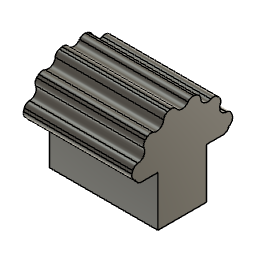
SMD-counter (Autodesk Fusion 360 archive; units mm, degrees)
design "roller"
Autodesk Fusion 360 part; units mm, degrees
note: some values were not read from the file. Set by a fixed rule: which face or edge a step refers to.
sketch "Sketch1" plane through (0, 0, 0) normal (0, 0, 1) x (1, 0, 0)
  line L0 (0, 0) -> (7.8, 0)
  line L1 (7.8, 0) -> (7.8, 3.5)
  line L2 (7.8, 3.5) -> (0, 3.5)
  line L3 (0, 3.5) -> (0, 0)
  dimension "d1" = 7.8
  dimension "d2" = 3.5
  constraint horizontal L0
  constraint vertical L1
  constraint horizontal L2
  constraint vertical L3
  constraint coincident L0.start L3.end
  measures "d1" distance of L0.start L0.end
  measures "d2" distance of L0.start L2.end
extrude "Extrude1" add sketch "Sketch1" along normal blind 3.6
sketch "Sketch2" plane through (7.8, 0, 0) normal (1, 0, 0) x (0, 1, 0)
  line L0 (0, 0) -> (3.5, 0)
  line L1 (3.5, 0) -> (3.5, 3.6)
  line L2 (3.5, 3.6) -> (0, 3.6)
  line L3 (0, 3.6) -> (0, 0)
  line L4 (-2, 3.6) -> (5.5, 3.6)
  arc A0 (5.5, 3.6) -> (-2, 3.6) centre (1.75, 3.4306) ccw
  dimension "d5" = 2
  dimension "d7" = 2
  constraint perpendicular L1 L4
  constraint collinear L2 L4
  measures "d5" distance of L3 L4.start
  measures "d7" distance of L1 L4.end
extrude "Extrude2" add sketch "Sketch2" against normal up to surface (7.8 mm away) contours L2 L4 A0
sketch "Sketch3" plane through (7.8, 0, 0) normal (1, 0, 0) x (0, 1, 0)
  line L0 (0, 0) -> (3.5, 0)
  line L1 (3.5, 0) -> (3.5, 3.6)
  line L2 (3.5, 3.6) -> (5.5, 3.6)
  arc A0 (5.5, 3.6) -> (-2, 3.6) centre (1.75, 3.4306) ccw
  line L3 (-2, 3.6) -> (0, 3.6)
  line L4 (0, 3.6) -> (0, 0)
  circle A1 centre (5.5, 3.6) radius 0.5
  circle A2 centre (4.9419, 5.4061) radius 0.5
  circle A3 centre (3.5744, 6.7112) radius 0.5
  circle A4 centre (1.7443, 7.1844) radius 0.5
  circle A5 centre (-0.0844, 6.7056) radius 0.5
  circle A6 centre (-1.4479, 5.3964) radius 0.5
  circle A7 centre (-2.0005, 3.5886) radius 0.5
  dimension "d11" = 1
  dimension "d13" = 175
  constraint coincident L2.end A0.start
  measures "d11" diameter of A1
extrude "Extrude3" cut sketch "Sketch3" against normal up to surface (7.8 mm away) contours A0 L3 A7 | L2 A0 A1 | A0 A6 | A0 A2 | A0 A5 | A0 A3 | A0 A4 picked at (-1.8378, 3.7013) picked at (5.3366, 3.7034) picked at (-1.3071, 5.3027) picked at (4.7922, 5.3274) picked at (0.0072, 6.5635) picked at (3.5029, 6.558) picked at (1.7326, 7.0157)
fillet "Fillet1" radius 0.4 14 edges at (3.9, -1.9462, 4.0856) (3.9, -1.6808, 4.9539) (3.9, -1.1583, 5.8039) (3.9, -0.5034, 6.4328) (3.9, 0.3671, 6.9204) (3.9, 1.2455, 7.1503) (3.9, 2.2432, 7.1518) (3.9, 3.1223, 6.9246) (3.9, 3.9943, 6.4396) (3.9, 4.6511, 5.8128) (3.9, 5.1762, 4.9643) (3.9, 5.4442, 4.0969) (3.9, 5, 3.6) (3.9, -1.5006, 3.6)
equation "d3 = ( 0.4 * 6 ) * 1 mm + 1.2 mm"

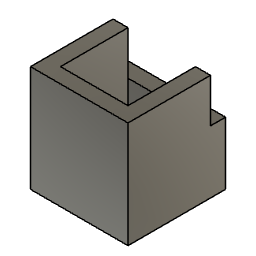
design "stopper"
Autodesk Fusion 360 part; units mm, degrees
sketch "Sketch1" plane through (0, 0, 0) normal (0, 0, 1) x (1, 0, 0)
  line L0 (0, 0) -> (7.8, 0)
  line L1 (7.8, 0) -> (7.8, 7.8)
  line L2 (7.8, 7.8) -> (0, 7.8)
  line L3 (0, 7.8) -> (0, 0)
  dimension "d1" = 7.8
  dimension "d2" = 7.8
  constraint horizontal L0
  constraint vertical L1
  constraint horizontal L2
  constraint vertical L3
  constraint coincident L0.start L3.end
  measures "d1" distance of L0.start L2.end
  measures "d2" distance of L1.end L2.end
extrude "Extrude1" add sketch "Sketch1" along normal blind 8.5
shell "Shell1" thickness 1.2 removed faces 1 at (2.6, 5.2, 8.5)
sketch "Sketch2" plane through (0, 7.8, 0) normal (0, 1, 0) x (-1, 0, 0)
  line L0 (-7.8, 0) -> (0, 0)
  line L1 (0, 0) -> (0, 8.5)
  line L2 (0, 8.5) -> (-7.8, 8.5)
  line L3 (-7.8, 8.5) -> (-7.8, 0)
  line L4 (-7.8, 8.5) -> (0, 8.5)
  line L5 (0, 8.5) -> (0, 5)
  line L6 (0, 5) -> (-7.8, 5)
  line L7 (-7.8, 5) -> (-7.8, 8.5)
  dimension "d6" = 3.5
  constraint horizontal L4
  constraint vertical L5
  constraint horizontal L6
  constraint vertical L7
  constraint coincident L1 L5.end
  constraint coincident L2.end L3.start
  measures "d6" distance of L2.end L6.end
extrude "Extrude2" cut sketch "Sketch2" against normal up to surface (1.2 mm away) contours L1 L2 L3 L4 L5 L6 L7
